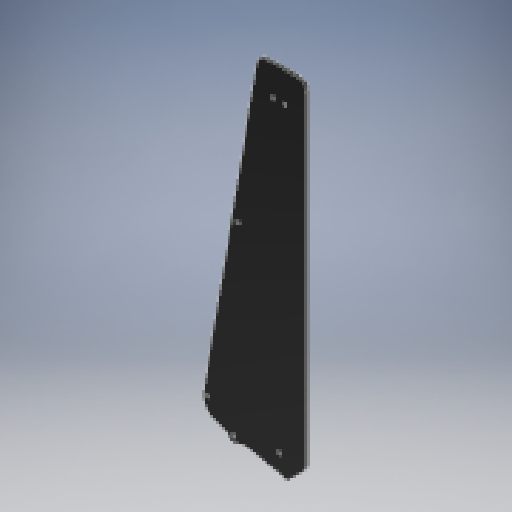
# Autodesk Inventor part: ChassisPolySides
Saved by Autodesk Inventor 2026.1 (Build 301233000, 233)
## iProperties
Created: 2025-09-20
Part Number: ChassisPolySides
Material: Acetal Resin, Black
Document SubType Name: Modeling
Designer: Teddy
Density: 1.425 g/cm^3
Appearance: Smooth - Black
Author: Teddy
Autodesk Inventor part; units mm, degrees
ref_plane "YZ Plane" through (0, 0, 0) normal (1, 0, 0) x (0, 1, 0)
ref_plane "XZ Plane" through (0, 0, 0) normal (0, 1, 0) x (-1, 0, 0)
ref_plane "Work Plane1" through (22.225, -368.3, 0) normal (0, 0, 1) x (1, 0, 0)
sketch "Sketch1" plane through (22.225, -368.3, 0) normal (0, 0, 1) x (1, 0, 0)
  line L0 (-22.225, 368.3) -> (-23.8125, 368.3) projected
  line L1 (1.5875, 368.3) -> (0, 368.3) projected
  line L2 (0.7938, -1.5875) -> (-32.5437, -1.5875) projected
  line L3 (-0.8984, -7.1348) -> (16.3738, 10.1374)
  line L4 (17.3038, 12.3825) -> (17.3038, 359.41)
  arc A0 (-3.8278, -7.9901) -> (-0.8984, -7.1348) centre (-3.1435, -4.8898) ccw
  arc A1 (16.3738, 10.1374) -> (17.3038, 12.3825) centre (14.1288, 12.3825) ccw
  line L5 (-3.8278, -7.9901) -> (-42.8925, 0.6322)
  line L6 (8.4138, 368.3) -> (-25.9965, 368.3)
  line L7 (-34.7595, 360.9075) -> (-91.6415, 28.0383)
  arc A2 (-91.5685, 28.3829) -> (-91.0646, 24.991) centre (-87.26, 27.2896) ccw construction
  arc A3 (-91.6415, 28.0383) -> (-79.9774, 8.8175) centre (-74.7339, 25.1491) ccw
  circle A4 centre (-11.1125, 12.7) radius 2.1844 projected
  circle A5 centre (-17.4625, 336.55) radius 2.1844 projected
  circle A6 centre (-4.7625, 336.55) radius 2.1844 projected
  arc A7 (-25.9965, 368.3) -> (-34.7595, 360.9075) centre (-25.9965, 359.41) ccw
  arc A8 (17.3038, 359.41) -> (8.4138, 368.3) centre (8.4138, 359.41) ccw
  circle A9 centre (-55.2671, 203.2) radius 6.35 construction
  circle A10 centre (-55.2671, 203.2) radius 2.286
  circle A11 centre (-87.26, 27.2896) radius 2.286 projected
  circle A12 centre (-59.2323, 4.2895) radius 2.286 projected
  arc A13 (-64.3491, 0.529) -> (-56.1738, -1.2754) centre (-59.2323, 4.2895) ccw
  arc A14 (-42.8925, 0.6322) -> (-56.1738, -1.2754) centre (-46.9984, -17.9701) ccw
  arc A15 (-64.3491, 0.529) -> (-75.5935, 7.8499) centre (-79.6994, -10.7524) ccw
  line L8 (-42.8925, 0.6322) -> (-75.5935, 7.8499) construction
  line L9 (-75.5935, 7.8499) -> (-79.9774, 8.8175)
  arc A16 (-65.4436, 5.6096) -> (-64.3491, 0.529) centre (-59.2323, 4.2895) ccw construction
  arc A17 (-56.1738, -1.2754) -> (-65.4436, 5.6096) centre (-59.2323, 4.2895) ccw construction
  point P0 (17.3038, 368.3)
  point P1 (-33.4962, 368.3)
  point P2 (-2.2536, -7.9375)
  point P3 (-23.0188, 368.3)
  point P4 (0.7938, 368.3)
  point P5 (0, 368.3)
  point P6 (-23.4578, 368.3)
  dimension "d0" = 16.51
  dimension "d1" = 3.175
  dimension "d3" = 50.8
  dimension "d4" = 6.35
  dimension "d5" = 45
  dimension "d6" = 8.89
  dimension "d7" = 4.572
  dimension "d8" = 165.1
  dimension "d11" = 12.7
  dimension "d12" = 19.05
  dimension "d13" = 19.05
  dimension "d14" = 13.97
  dimension "d15" = 12.7
  constraints: 22 point on circle, 21 tangent, 14 end point, 12 centre point, 6 point on line, 3 coincident, 2 equal radius, 1 horizontal, 1 horizontal alignment, 1 midpoint, 1 perpendicular, 1 other
  measures "d0" distance from line of L2.start L4
  measures "d1" radius of A0
  measures "d3" distance of point (17.304, 368.3) point (-33.496, 368.3)
  measures "d4" distance from line of L2 point (-2.254, -7.938)
  measures "d5" angle of L4 L3
  measures "d6" radius of A7
  measures "d7" diameter of A10
  measures "d8" distance from line of L6 A9.centre
  measures "d11" diameter of A13
  measures "d12" radius of A14
  measures "d13" radius of A15
  measures "d14" distance from line of L2 L4.start
  measures "d15" diameter of A9
extrude "Extrusion1" add sketch "Sketch1" along normal blind 3.175
body "Solid1"
